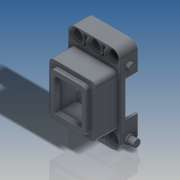
# Autodesk Inventor part: 10825-LtBluishGray
Saved by Autodesk Inventor 2016 SP2 (Build 200236200, 236)
## iProperties
Created: 2015-09-01
Part Number: 10825-LtBluishGray
Material: ABS Plastic
Document SubType Name: Modeling
Designer: D. Kohfeld
Density: 1.06 g/cm^3
Appearance: LtBluishGray
Mass: 3.39541 g
Surface Area: 55.5957 cm^2
Volume: 3.20321 cm^3
Author: D. Kohfeld
Autodesk Inventor part; units mm, degrees
ref_plane "YZ Plane" through (0, 0, 0) normal (1, 0, 0) x (0, 1, 0)
ref_plane "XZ Plane" through (0, 0, 0) normal (0, 1, 0) x (-1, 0, 0)
ref_plane "XY Plane" through (0, 0, 0) normal (0, 0, 1) x (1, 0, 0)
sketch "Sketch2" plane through (0, 0, 0) normal (0, 0, 1) x (1, 0, 0)
  line L0 (-11.6, 16) -> (-11.6, -16)
  arc A0 (-11.6, -16) -> (-8, -19.6) centre (-8, -16) ccw
  line L1 (-8, -19.6) -> (8, -19.6)
  arc A1 (8, -19.6) -> (11.6, -16) centre (8, -16) ccw
  line L2 (11.6, -16) -> (11.6, 16)
  arc A2 (11.6, 16) -> (8, 19.6) centre (8, 16) ccw
  line L3 (8, 19.6) -> (-8, 19.6)
  arc A3 (-8, 19.6) -> (-11.6, 16) centre (-8, 16) ccw
  circle A4 centre (-8, 16) radius 3.1
  circle A5 centre (-8, 16) radius 2.4
  circle A6 centre (8, 16) radius 3.1
  circle A7 centre (8, 16) radius 2.4
  circle A8 centre (0, 16) radius 3.1
  circle A9 centre (0, 16) radius 2.4
  circle A10 centre (-8, -16) radius 3.1
  circle A11 centre (-8, -16) radius 2.4
  circle A12 centre (0, -16) radius 2.4
  circle A13 centre (0, -16) radius 3.1
  circle A14 centre (8, -16) radius 3.1
  circle A15 centre (8, -16) radius 2.4
  line L4 (-8, 16) -> (0, 16) construction
  line L5 (0, 16) -> (8, 16) construction
  line L6 (8, 16) -> (8, -16) construction
  line L7 (-5.04, 7.36) -> (5.04, 7.36)
  line L8 (6, 6.4) -> (6, -7.2)
  line L9 (6, -7.2) -> (-6, -7.2)
  line L10 (-6, -7.2) -> (-6, 6.4)
  line L11 (-6, 9.6) -> (6, 9.6)
  line L12 (8, 7.6) -> (8, -7.6)
  line L13 (6, -9.6) -> (-6, -9.6)
  line L14 (-8, -7.6) -> (-8, 7.6)
  line L15 (-8.4, 11.6) -> (8.4, 11.6)
  line L16 (10.4, 9.6) -> (10.4, -9.6)
  line L17 (8.4, -11.6) -> (-8.4, -11.6)
  line L18 (-10.4, -9.6) -> (-10.4, 9.6)
  arc A16 (-5.04, 7.36) -> (-6, 6.4) centre (-5.04, 6.4) ccw
  arc A17 (6, 6.4) -> (5.04, 7.36) centre (5.04, 6.4) ccw
  arc A18 (-6, 9.6) -> (-8, 7.6) centre (-6, 7.6) ccw
  arc A19 (-8, -7.6) -> (-6, -9.6) centre (-6, -7.6) ccw
  arc A20 (6, -9.6) -> (8, -7.6) centre (6, -7.6) ccw
  arc A21 (8, 7.6) -> (6, 9.6) centre (6, 7.6) ccw
  arc A22 (-8.4, 11.6) -> (-10.4, 9.6) centre (-8.4, 9.6) ccw
  arc A23 (-10.4, -9.6) -> (-8.4, -11.6) centre (-8.4, -9.6) ccw
  arc A24 (8.4, -11.6) -> (10.4, -9.6) centre (8.4, -9.6) ccw
  arc A25 (10.4, 9.6) -> (8.4, 11.6) centre (8.4, 9.6) ccw
  line L19 (-5.4544, 18.5456) -> (-2.5456, 18.5456)
  line L20 (-5.4544, 13.4544) -> (-2.5456, 13.4544)
  line L21 (2.5456, 18.5456) -> (5.4544, 18.5456)
  line L22 (2.5456, 13.4544) -> (5.4544, 13.4544)
  line L23 (-5.4544, -13.4544) -> (-2.5456, -13.4544)
  line L24 (-5.4544, -18.5456) -> (-2.5456, -18.5456)
  line L25 (2.5456, -13.4544) -> (5.4544, -13.4544)
  line L26 (2.5456, -18.5456) -> (5.4544, -18.5456)
  arc A26 (-5.4544, 13.4544) -> (-5.4544, 18.5456) centre (-8, 16) ccw
  arc A27 (-2.5456, 18.5456) -> (-2.5456, 13.4544) centre (0, 16) ccw
  arc A28 (2.5456, 13.4544) -> (2.5456, 18.5456) centre (0, 16) ccw
  arc A29 (5.4544, 18.5456) -> (5.4544, 13.4544) centre (8, 16) ccw
  arc A30 (-5.4544, -18.5456) -> (-5.4544, -13.4544) centre (-8, -16) ccw
  arc A31 (-2.5456, -13.4544) -> (-2.5456, -18.5456) centre (0, -16) ccw
  arc A32 (2.5456, -18.5456) -> (2.5456, -13.4544) centre (0, -16) ccw
  arc A33 (5.4544, -13.4544) -> (5.4544, -18.5456) centre (8, -16) ccw
  line L27 (8, 16) -> (5.4544, 18.5456) construction
  point P0 (0, 0)
  point P1 (0, 19.6)
  point P2 (-11.6, 0)
  point P3 (8, 0)
  point P4 (0, 7.36)
  point P5 (0, 9.6)
  point P6 (0, 11.6)
  point P7 (-8, 0)
  point P8 (-10.4, 0)
  dimension "d0" = 3.6
  dimension "d2" = 4.8
  dimension "d3" = 6.2
  dimension "d4" = 8
  dimension "d5" = 32
  dimension "d6" = 0.96
  dimension "d7" = 2
  dimension "d8" = 14.56
  dimension "d9" = 19.2
  dimension "d10" = 23.2
  dimension "d11" = 12
  dimension "d12" = 16
  dimension "d13" = 2.4
  dimension "d14" = 20.8
  dimension "d15" = 45
  constraints: 56 end point, 44 point on circle, 34 centre point, 29 equal radius, 28 tangent, 18 coincident, 15 horizontal, 8 equal length, 8 midpoint, 7 vertical alignment, 6 horizontal alignment, 6 parallel, 3 perpendicular, 3 vertical
  measures "d0" radius of A2
  measures "d2" diameter of A7
  measures "d3" diameter of A6
  measures "d4" distance of L4.end L5.end
  measures "d5" distance of L5.end L6.end
  measures "d6" radius of A16
  measures "d7" radius of A18
  measures "d8" distance between parallel lines of L9 L7
  measures "d9" distance between parallel lines of L11 L13
  measures "d10" distance between parallel lines of L17 L15
  measures "d11" distance between parallel lines of L8 L10
  measures "d12" distance between parallel lines of L12 L14
  measures "d13" distance between parallel lines of L13 L9
  measures "d14" distance between parallel lines of L16 L18
  measures "d15" angle of L27 L21
extrude "Extrusion1" add sketch "Sketch2" against normal blind 8 contours A3 L3 A2 L2 A1 L1 A0 L0 | A4 | A6 | A8 | A10 | A13 | A14 | L11 A21 L12 A20 L13 A19 L14 A18 | L15 A25 L16 A24 L17 A23 L18 A22 | L19 A27 L20 A26 | L21 A29 L22 A28 | L23 A31 L24 A30 | L25 A33 L26 A32
extrude "Extrusion2" cut sketch "Sketch2" against normal blind 0.8 contours A4 | A6 | A8 | A10 | A13 | A14
extrude "Extrusion3" cut sketch "Sketch2" against normal blind 6.4 contours L19 A27 L20 A26 | L21 A29 L22 A28 | L23 A31 L24 A30 | L25 A33 L26 A32
extrude "Extrusion4" add sketch "Sketch2" along normal blind 9.6 contours L11 A21 L12 A20 L13 A19 L14 A18 | L15 A25 L16 A24 L17 A23 L18 A22
extrude "Extrusion5" add sketch "Sketch2" along normal blind 11.6 contours L11 A21 L12 A20 L13 A19 L14 A18
sketch "Sketch3" plane through (0, 0, -8) normal (0, 0, -1) x (-1, 0, 0)
  circle A0 centre (-8, -16) radius 2.4 projected
  circle A1 centre (0, -16) radius 2.4 projected
  circle A2 centre (8, -16) radius 2.4 projected
  circle A3 centre (0, 16) radius 2.4 projected
  circle A4 centre (-8, 16) radius 2.4 projected
  circle A5 centre (8, 16) radius 2.4 projected
  line L0 (11.6, -16) -> (11.6, 16) projected
  arc A6 (11.6, 16) -> (8, 19.6) centre (8, 16) ccw projected
  arc A7 (-8, 19.6) -> (-11.6, 16) centre (-8, 16) ccw projected
  line L1 (-11.6, 16) -> (-11.6, -16) projected
  arc A8 (-11.6, -16) -> (-8, -19.6) centre (-8, -16) ccw projected
  arc A9 (8, -19.6) -> (11.6, -16) centre (8, -16) ccw projected
  line L2 (-10.4, 12.4) -> (10.4, 12.4)
  line L3 (10.4, 12.4) -> (10.4, -12.4)
  line L4 (10.4, -12.4) -> (-10.4, -12.4)
  line L5 (-10.4, -12.4) -> (-10.4, 12.4)
  line L6 (-9.2, 10.4) -> (9.2, 10.4)
  line L7 (9.2, 10.4) -> (9.2, -10.4)
  line L8 (9.2, -10.4) -> (-9.2, -10.4)
  line L9 (-9.2, -10.4) -> (-9.2, 10.4)
  line L10 (-10.4, 8) -> (-11.6, 8)
  line L11 (-10.4, -8) -> (-11.6, -8)
  line L12 (10.4, -8) -> (11.6, -8)
  line L13 (10.4, 8) -> (11.6, 8)
  circle A10 centre (-8, 16) radius 3.1
  circle A11 centre (0, 16) radius 3.1
  circle A12 centre (8, 16) radius 3.1
  circle A13 centre (-8, -16) radius 3.1
  circle A14 centre (0, -16) radius 3.1
  circle A15 centre (8, -16) radius 3.1
  point P0 (0, 0)
  point P1 (0, 10.4)
  point P2 (0, 12.4)
  point P3 (-9.2, 0)
  point P4 (-10.4, 0)
  dimension "d26" = 24.8
  dimension "d27" = 16
  dimension "d28" = 20.8
  dimension "d29" = 18.4
  dimension "d30" = 20.8
  dimension "d31" = 4.4
  dimension "d32" = 6.2
  constraints: 24 end point, 8 point on line, 6 centre point, 6 coincident, 6 horizontal, 5 equal radius, 4 horizontal alignment, 4 midpoint, 4 parallel, 2 perpendicular, 2 vertical alignment
  measures "d26" distance of L2.end L3.end
  measures "d27" distance between parallel lines of L12 L13
  measures "d28" distance of L2.start L2.end
  measures "d29" distance between parallel lines of L7 L9
  measures "d30" distance between parallel lines of L8 L6
  measures "d31" distance between parallel lines of L2 L10
  measures "d32" diameter of A12
extrude "Extrusion6" cut sketch "Sketch3" against normal blind 0.8 contours A10 | A11 | A12 | A13 | A14 | A15
extrude "Extrusion7" cut sketch "Sketch3" against normal blind 5.6 contours L12 L3 L13 L0 | L11 L1 L10 L5
extrude "Extrusion8" cut sketch "Sketch3" against normal blind 6.8 contours L3 L4 L5 L2
extrude "Extrusion9" cut sketch "Sketch3" against normal blind 17.2 contours L6 L7 L8 L9
sketch "Sketch4" plane through (11.6, -16, 0) normal (1, 0, 0) x (0, 0, -1)
  line L0 (0, 0) -> (8, 0) construction
  line L1 (8, 8) -> (8, 0) projected
  circle A0 centre (4, 28.4) radius 1.6
  circle A1 centre (4, 0) radius 2
  circle A2 centre (4, 0) radius 1.6
  point P0 (0, 16)
  dimension "d41" = 3.2
  dimension "d42" = 4
  dimension "d43" = 4
  dimension "d44" = 28.4
  constraints: 3 centre point, 1 coincident, 1 equal radius, 1 midpoint, 1 vertical alignment
  measures "d41" diameter of A0
  measures "d42" diameter of A1
  measures "d43" distance from line of L1 A1.centre
  measures "d44" distance of A1.centre A0.centre
extrude "Extrusion10" add sketch "Sketch4" along normal blind 1.6 contours A0
extrude "Extrusion11" add sketch "Sketch4" along normal blind 0.8 contours A1
extrude "Extrusion12" add sketch "Sketch4" against normal up to surface contours A1 | A2
extrude "Extrusion13" add sketch "Sketch4" along normal blind 3.6 contours A2
mirror "Mirror1" about plane through (0, 0, 0) normal (1, 0, 0) of "Extrusion10", "Extrusion11", "Extrusion12", "Extrusion13"
fillet "Fillet1" radius 0.1 78 edges at (-10.5456, -18.5456, 0) (0, -19.6, 0) (10.5456, -18.5456, 0) (11.6, 0, 0) (10.5456, 18.5456, 0) (0, 19.6, 0) (-10.5456, 18.5456, 0) (-11.6, 0, 0) (-9.8142, 11.0142, 9.6) (-10.4, 0, 9.6) (-9.8142, -11.0142, 9.6) (0, -11.6, 9.6) (9.8142, -11.0142, 9.6) (10.4, 0, 9.6) (9.8142, 11.0142, 9.6) (0, 11.6, 9.6) (-7.4142, 9.0142, 11.6) (-8, 0, 11.6) (-7.4142, -9.0142, 11.6) (0, -9.6, 11.6) (7.4142, -9.0142, 11.6) (8, 0, 11.6) (7.4142, 9.0142, 11.6) (0, 9.6, 11.6) (-5.7188, 7.0788, 11.6) (0, 7.36, 11.6) (5.7188, 7.0788, 11.6) (6, -0.4, 11.6) (-6, -0.4, 11.6) (0, -7.2, 11.6) (0, -7.2, 9.2) (-5.7188, 7.0788, 9.2) (0, 7.36, 9.2) (5.7188, 7.0788, 9.2) (6, -0.4, 9.2) (-6, -0.4, 9.2) (-9.2, 0, -1.2) (0, -10.4, -1.2) (11.6, 0, -2.4) (11.6, -8, -5.2) (10.4, -8, -5.2) (11, -8, -8) (10.5456, -18.5456, -8) (0, -19.6, -8) (-10.5456, -18.5456, -8) (-11.6, -12, -8) (11.6, -12, -8) (10.4, -10.2, -8) (0, -12.4, -8) (12.4, -16, -2) (15.2, -16, -2.4) (13.2, 12.4, -2.4) (11.6, 12, -8) (0, 19.6, -8) (-10.5456, 18.5456, -8) (-11.6, 12, -8) (10.5456, 18.5456, -8) (-12.4, -16, -2) (-15.2, -16, -2.4) (-13.2, 12.4, -2.4) (0, 12.4, -8) (10.4, 10.2, -8) (11, 8, -8) (10.4, 8, -5.2) (11.6, 8, -5.2) (10.4, 0, -2.4) (-10.4, 10.2, -8) (-11.6, 8, -5.2) (-11, 8, -8) (-10.4, 8, -5.2) (-11.6, 0, -2.4) (-10.4, 0, -2.4) (-11.6, -8, -5.2) (-10.4, -8, -5.2) (-11, -8, -8) (-10.4, -10.2, -8) (0, 10.4, -1.2) (9.2, 0, -1.2)
fillet "Fillet1" radius 0.4 16 edges at (-5.4544, 18.5456, -3.2) (-2.5456, 18.5456, -3.2) (-5.4544, 13.4544, -3.2) (-2.5456, 13.4544, -3.2) (2.5456, 13.4544, -3.2) (5.4544, 13.4544, -3.2) (2.5456, 18.5456, -3.2) (5.4544, 18.5456, -3.2) (2.5456, -18.5456, -3.2) (5.4544, -18.5456, -3.2) (-2.5456, -18.5456, -3.2) (-5.4544, -18.5456, -3.2) (-5.4544, -13.4544, -3.2) (-2.5456, -13.4544, -3.2) (2.5456, -13.4544, -3.2) (5.4544, -13.4544, -3.2)
equation "\"d0\" = 0.5 * tlad"
equation "\"d2\" = tpd"
equation "\"d3\" = tsd"
equation "\"d4\" = lu"
equation "\"d5\" = 4 * lu"
equation "\"d12\" = 2 * lu"
equation "\"d16\" = lu"
equation "\"d18\" = tsl"
equation "\"d27\" = 2 * lu"
equation "\"d32\" = tsd"
equation "\"d33\" = tsl"
equation "\"d41\" = rd"
equation "\"d45\" = wall"
equation "\"d53\" = lf"
equation "\"d54\" = tf"
equation "\"tlad\" = 7.2"
equation "\"tpd\" = 4.8"
equation "\"tsd\" = 6.2"
equation "\"lu\" = 8"
equation "\"tsl\" = 0.8"
equation "\"rd\" = 3.2"
equation "\"wall\" = 1.6"
equation "\"lf\" = 0.1"
equation "\"tf\" = 0.4"
body "Solid1"
